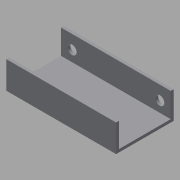
# Autodesk Inventor part: 3in C-Channel (TopPlate Supports Rear)
Saved by Autodesk Inventor 2013 (Build 170138000, 138)
## iProperties
Created: 2013-01-27
Part Number: 3in C-Channel (TopPlate Supports Rear)
Material: Aluminum 6061
Document SubType Name: Modeling
Designer: Naphat
Density: 1 g/cm^3
Author: Naphat
Autodesk Inventor part; units mm, degrees
ref_plane "YZ Plane" through (0, 0, 0) normal (1, 0, 0) x (0, 1, 0)
ref_plane "XZ Plane" through (0, 0, 0) normal (0, 1, 0) x (-1, 0, 0)
ref_plane "XY Plane" through (0, 0, 0) normal (0, 0, 1) x (1, 0, 0)
sketch "Sketch1" plane through (0, 0, 0) normal (1, 0, 0) x (0, 1, 0)
  line L0 (0, 0) -> (0, -40)
  line L1 (0, -40) -> (19, -40)
  line L2 (19, -40) -> (19, -38)
  line L3 (0, 0) -> (19, 0)
  line L4 (19, 0) -> (19, -2)
  line L5 (0, -20) -> (2, -20) construction
  line L6 (19, -2) -> (2, -2)
  line L7 (2, -2) -> (2, -38)
  line L8 (2, -38) -> (19, -38)
  dimension "d0" = 40
  dimension "d1" = 19
  dimension "d2" = 2
  dimension "d3" = 2
  dimension "d4" = 2
  constraints: 18 end point, 6 perpendicular, 2 parallel, 1 midpoint, 1 vertical
  measures "d0" distance of L0.start L0.end
  measures "d1" distance of L0.end L1.end
  measures "d2" distance of L1.end L2.end
  measures "d3" distance of L3.end L4.end
  measures "d4" distance of L5.start L5.end
extrude "Extrusion1" add sketch "Sketch1" along normal blind 76.2
sketch "Sketch4" plane through (0, 0, -40) normal (0, 0, -1) x (-1, 0, 0)
  line L0 (-76.2, 9.5) -> (-68.58, 9.5) construction
  line L1 (-76.2, 9.5) -> (-68.58, 9.5) construction
  circle A0 centre (-68.58, 9.5) radius 3.175
  line L2 (0, 0) -> (0, 19) projected
  line L3 (0, 0) -> (-76.2, 0) projected
  line L4 (0, 9.5) -> (-7.62, 9.5) construction
  circle A1 centre (-7.62, 9.5) radius 3.175
  dimension "d11" = 7.62
  dimension "d12" = 6.35
  dimension "d16" = 7.62
  dimension "d17" = 6.35
  constraints: 6 end point, 2 centre point, 2 coincident, 1 collinear, 1 horizontal, 1 midpoint, 1 parallel
  measures "d11" distance of L0.start L0.end
  measures "d12" diameter of A0
  measures "d16" distance of L4.start L4.end
  measures "d17" diameter of A1
extrude "Extrusion4" cut sketch "Sketch4" against normal blind 25.4
body "Solid1"
